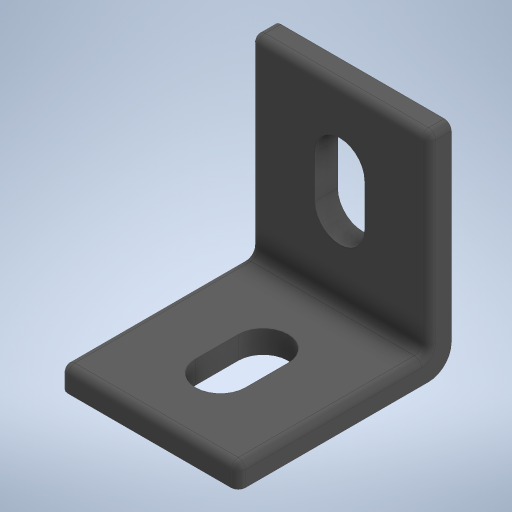
# Autodesk Inventor part: 안쪽브라켓
Saved by Autodesk Inventor 2024 (Build 280153000, 153)
## iProperties
Created: 2024-04-09
Part Number: 안쪽브라켓
Material: 일반
Document SubType Name: Modeling
Designer: kkamin5
Density: 1 g/cm^3
Appearance: 기본값
Author: kkamin5
Autodesk Inventor part; units mm, degrees
ref_plane "YZ Plane" through (0, 0, 0) normal (1, 0, 0) x (0, 1, 0)
ref_plane "XZ Plane" through (0, 0, 0) normal (0, 1, 0) x (-1, 0, 0)
sketch "스케치1" plane through (0, 0, 0) normal (1, 0, 0) x (0, 1, 0)
  line L0 (0, 10) -> (0, 30)
  line L1 (0, 30) -> (3.2, 30)
  line L2 (3.2, 30) -> (3.2, 3.2)
  line L3 (3.2, 3.2) -> (30, 3.2)
  line L4 (30, 3.2) -> (30, 0)
  line L5 (30, 0) -> (0, 0)
  line L6 (0, 0) -> (0, 10)
  dimension "d2" = 3.2
  dimension "d3" = 26.8
  dimension "d4" = 26.8
  dimension "d5" = 90
  dimension "d6" = 3.2
  dimension "d13" = 90
  dimension "d14" = 10
  constraints: 14 end point, 4 perpendicular, 1 coincident, 1 collinear, 1 point on line, 1 vertical
  measures "d2" distance of L0.end L1.end
  measures "d3" distance of L1.end L2.end
  measures "d4" distance of L2.end L3.end
  measures "d5" angle of L3 L2
  measures "d6" distance of L3.end L4.end
  measures "d13" angle of L4 L5
  measures "d14" distance of L5.end L0.start
extrude "돌출1" add sketch "스케치1" along normal mid plane 25
sketch "스케치2" plane through (-12.5, 3.2, 30) normal (0, 1, 0) x (1, 0, 0)
  line L0 (12.5, 10) -> (12.5, 16) construction
  line L1 (16, 10) -> (16, 16)
  line L2 (9, 16) -> (9, 10)
  arc A0 (9, 10) -> (16, 10) centre (12.5, 10) ccw
  arc A1 (16, 16) -> (9, 16) centre (12.5, 16) ccw
  line L3 (0, 0) -> (25, 0) projected
  line L4 (0, 0) -> (0, 26.8) projected
  point P0 (12.5, 30)
  point P1 (12.5, 13)
  point P2 (0, 13.4)
  dimension "d10" = 6
  dimension "d11" = 7
  dimension "d12" = 10
  dimension "d15" = 12.5
  constraints: 8 end point, 4 point on circle, 4 tangent, 2 centre point, 2 midpoint, 1 parallel, 1 vertical
  measures "d10" distance of L0.start L0.end
  measures "d11" diameter of A1
  measures "d12" distance from line of L3 L0.start
  measures "d15" horizontal distance of point (0, 13.4) point (12.5, 13)
extrude "돌출2" cut sketch "스케치2" against normal through all
ref_plane "작업 평면1" through (-12.5, 3.2, 3.2) normal (0, 0.7071, -0.7071) x (-1, 0, 0)
mirror "미러1" about plane through (-12.5, 3.2, 3.2) normal (0, 0.7071, -0.7071) of "돌출2"
fillet "모깎기2" radius 1 11 edges at (12.5, 16.6, 3.2) (0, 30, 3.2) (-12.5, 16.6, 3.2) (12.5, 3.2, 16.6) (0, 3.2, 30) (-12.5, 3.2, 16.6) (0, 3.2, 3.2) (12.5, 30, 1.6) (-12.5, 30, 1.6) (-12.5, 1.6, 30) (12.5, 1.6, 30)
fillet "모깎기3" radius 3.2 1 edges at (0, 0, 0)
